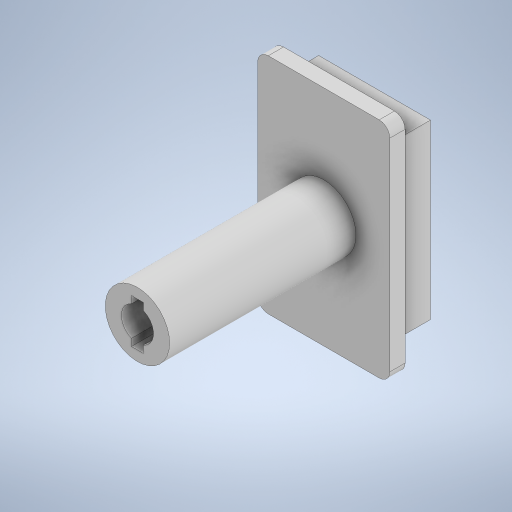
# Autodesk Inventor part: reset_switch
Saved by Autodesk Inventor 2024 (Build 280153000, 153)
## iProperties
Created: 2023-06-19
Part Number: reset_switch
Material: Generic
Document SubType Name: Modeling
Designer: jconvertino
Density: 1 g/cm^3
Appearance: Default
Author: jconvertino
Autodesk Inventor part; units mm, degrees
ref_plane "YZ Plane" through (0, 0, 0) normal (1, 0, 0) x (0, 1, 0)
ref_plane "XZ Plane" through (0, 0, 0) normal (0, 1, 0) x (-1, 0, 0)
ref_plane "XY Plane" through (0, 0, 0) normal (0, 0, 1) x (1, 0, 0)
sketch "Sketch1" plane through (0, 0, 0) normal (0, 0, 1) x (1, 0, 0)
  line L0 (0, 0) -> (16.764, 0)
  line L1 (16.764, 0) -> (16.764, 25.908)
  line L2 (16.764, 25.908) -> (0, 25.908)
  line L3 (0, 25.908) -> (0, 0)
  dimension "d0" = 16.764
  dimension "d1" = 25.908
  constraints: 8 end point, 2 parallel, 1 horizontal, 1 perpendicular
  measures "d0" distance of L1.end L2.end
  measures "d1" distance of L0.end L1.end
extrude "Extrusion1" add sketch "Sketch1" along normal blind 5.334
sketch "Sketch2" plane through (0, 0, 5.334) normal (0, 0, 1) x (1, 0, 0)
  line L0 (-1.524, 29.718) -> (18.288, 29.718)
  line L1 (18.288, 29.718) -> (18.288, -3.81)
  line L2 (18.288, -3.81) -> (-1.524, -3.81)
  line L3 (-1.524, -3.81) -> (-1.524, 29.718)
  line L4 (16.764, 25.908) -> (0, 25.908) projected
  line L5 (0, 0) -> (16.764, 0) projected
  line L6 (0, 25.908) -> (0, 0) projected
  line L7 (16.764, 0) -> (16.764, 25.908) projected
  dimension "d4" = 3.81
  dimension "d5" = 3.81
  dimension "d6" = 1.524
  dimension "d7" = 1.524
  constraints: 8 end point, 2 parallel, 1 horizontal, 1 perpendicular
  measures "d4" distance between parallel lines of L4 L0
  measures "d5" distance between parallel lines of L2 L5
  measures "d6" distance between parallel lines of L6 L3
  measures "d7" distance between parallel lines of L1 L7
extrude "Extrusion2" add sketch "Sketch2" along normal blind 2.286 contours L0 L1 L2 L3 | L7 L5 L6 L4
sketch "Sketch3" plane through (0, 0, 7.62) normal (0, 0, 1) x (1, 0, 0)
  circle A0 centre (8.382, 12.954) radius 4.826
  line L0 (18.288, 29.718) -> (-1.524, 29.718) projected
  line L1 (-1.524, -3.81) -> (18.288, -3.81) projected
  line L2 (-1.524, 29.718) -> (-1.524, -3.81) projected
  line L3 (18.288, -3.81) -> (18.288, 29.718) projected
  point P0 (0, 0)
  dimension "d10" = 16.764
  dimension "d11" = 16.764
  dimension "d12" = 9.906
  dimension "d13" = 9.906
  dimension "d14" = 9.652
  constraints: 1 centre point
  measures "d10" distance from line of L0 A0.centre
  measures "d11" distance from line of L1 A0.centre
  measures "d12" distance from line of L2 A0.centre
  measures "d13" distance from line of L3 A0.centre
  measures "d14" diameter of A0
extrude "Extrusion3" add sketch "Sketch3" along normal blind 27.94 contours A0
sketch "Sketch4" plane through (8.382, 12.954, 35.56) normal (0, 0, 1) x (1, 0, 0)
  circle A0 centre (0, 0) radius 2.413
  line L0 (-0.889, 3.302) -> (0.889, 3.302)
  line L1 (0.889, 3.302) -> (0.889, -3.302)
  line L2 (0.889, -3.302) -> (-0.889, -3.302)
  line L3 (-0.889, -3.302) -> (-0.889, 3.302)
  circle A1 centre (0, 0) radius 4.826 projected
  point P0 (-8.382, -12.954)
  point P1 (-0.889, 0)
  point P2 (0.889, 0)
  point P3 (-0.889, -2.2433)
  point P4 (0.889, -2.2433)
  point P5 (0.889, 2.2433)
  point P6 (-0.889, 2.2433)
  dimension "d17" = 4.826
  dimension "d18" = 0.889
  dimension "d19" = 0.889
  dimension "d20" = 3.302
  dimension "d21" = 3.302
  constraints: 8 end point, 2 midpoint, 2 parallel, 1 centre point, 1 concentric, 1 horizontal, 1 perpendicular
  measures "d17" diameter of A0
  measures "d18" distance of point (-0.889, 0) A0.centre
  measures "d19" distance of point (0.889, 0) A0.centre
  measures "d20" distance from line of L0 A0.centre
  measures "d21" distance from line of L2 A0.centre
extrude "Extrusion4" cut sketch "Sketch4" against normal blind 27.94 contours A0 L1 | L1 A0 L3 | A0 L3 L0 L1 | L1 L2 L3 A0 | L3 A0
sketch "Sketch5" plane through (0, 0, 0) normal (0, 0, -1) x (-1, 0, 0)
  arc A0 (-7.493, 10.7107) -> (-7.493, 15.1973) centre (-8.382, 12.954) ccw projected
  circle A1 centre (-8.382, 12.954) radius 6.0325
  point P0 (0, 0)
  dimension "d24" = 12.065
  constraints: 1 centre point, 1 coincident
  measures "d24" diameter of A1
extrude "Extrusion5" cut sketch "Sketch5" against normal blind 1.5875
fillet "Fillet1" radius 3.175 1 edges at (14.4145, 12.954, 1.5875)
fillet "Fillet3" radius 1.5875 4 edges at (-1.524, 29.718, 6.477) (-1.524, -3.81, 6.477) (18.288, 29.718, 6.477) (18.288, -3.81, 6.477)
body "Solid1"
